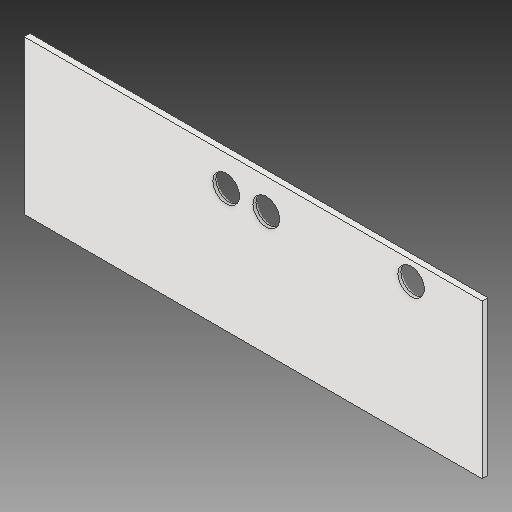
# Autodesk Inventor part: back_plate
Saved by Autodesk Inventor 2017 (Build 210142000, 142)
## iProperties
Created: 2018-01-15
Part Number: back_plate
Material: Generic
Document SubType Name: Modeling
Designer: Mitch
Density: 1 g/cm^3
Appearance: White
Author: Mitch
Autodesk Inventor part; units mm, degrees
ref_plane "YZ Plane" through (0, 0, 0) normal (1, 0, 0) x (0, 1, 0)
ref_plane "XZ Plane" through (0, 0, 0) normal (0, 1, 0) x (-1, 0, 0)
ref_plane "XY Plane" through (0, 0, 0) normal (0, 0, 1) x (1, 0, 0)
sketch "Sketch1" plane through (0, 0, 0) normal (0, 0, 1) x (1, 0, 0)
  line L0 (0, 0) -> (130.3782, 0)
  line L1 (130.3782, 0) -> (130.3782, 43.815)
  line L2 (130.3782, 43.815) -> (0, 43.815)
  line L3 (0, 43.815) -> (0, 0)
  dimension "d0" = 130.3782
  dimension "d1" = 43.815
  constraints: 8 end point, 2 parallel, 1 horizontal, 1 perpendicular
  measures "d0" distance of L2.end L1.end
  measures "d1" distance of L1.end L0.end
extrude "Extrusion1" add sketch "Sketch1" along normal blind 1.651
sketch "Sketch2" plane through (0, 0, 0) normal (0, 0, -1) x (-1, 0, 0)
  circle A0 centre (-110.162, 38.5548) radius 3.25 projected
  circle A1 centre (-68.9426, 35.1048) radius 1.75 projected
  circle A2 centre (-57.5127, 35.1048) radius 1.75 projected
  circle A3 centre (-110.162, 38.5548) radius 3.758
  circle A4 centre (-68.9426, 35.1048) radius 3.8074
  circle A5 centre (-57.5127, 35.1048) radius 3.8074
  point P0 (0, 0)
  dimension "d4" = 0.508
  dimension "d5" = 3.5
  dimension "d6" = 2.0574
  dimension "d7" = 2.0574
  constraints: 3 centre point
  measures "d4" radial gap between concentric circles of A0 A3
  measures "d5" diameter of A1
  measures "d6" radial gap between concentric circles of A1 A4
  measures "d7" radial gap between concentric circles of A2 A5
extrude "Extrusion2" cut sketch "Sketch2" against normal blind 1.651 contours A0 | A1 | A2 | A3 | A4 | A5
fillet "Fillet1" radius 0.7937 3 edges at (113.92, 38.5548, 0) (72.75, 35.1048, 0) (61.3201, 35.1048, 0)
body "Solid1"
